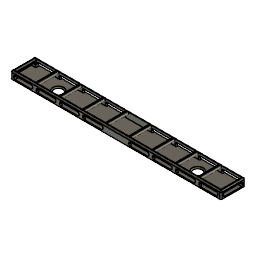
Velcro tie holder (Autodesk Fusion 360 design; units mm, degrees)
part number: 2026-08-08-13-01-59-133
Autodesk Fusion 360 part; units mm, degrees
note: some values were not read from the file. Set by a fixed rule: which face or edge a step refers to.
sketch "Sketch1" plane through (0, 0, 0) normal (0, 0, 1) x (1, 0, 0)
  line L0 (0, 0) -> (20, 0)
  line L1 (20, 0) -> (20, 20)
  line L2 (20, 20) -> (0, 20)
  line L3 (0, 20) -> (0, 0)
  dimension "d1" = 20
  dimension "d2" = 20
  constraint horizontal L0
  constraint vertical L1
  constraint horizontal L2
  constraint vertical L3
  constraint coincident L0.start L3.end
  measures "d1" distance of L0.start L0.end
  measures "d2" distance of L0.start L2.end
extrude "Extrude1" add sketch "Sketch1" along normal blind 1 makes body 1
extrude "Extrude2" add 1 faces at (6.6667, 13.3333, 1) along direction (0, 0, 1) blind 4 thin wall 1 inside on bodies 1 bodies 1
shell "Shell1" thickness 1 removed faces 2 at (6.6667, 0, 1.6667) at (7, 1, 2.3333) on bodies 1
shell "Shell2" thickness 1 removed faces 2 at (20, 6.6667, 1.6667) at (19, 13, 3.3333) on bodies 1
shell "Shell3" thickness 1 removed faces 2 at (0, 13.3333, 1.6667) at (1, 13, 3.3333) on bodies 1
shell "Shell4" thickness 1 removed faces 2 at (13.3333, 20, 1.6667) at (7, 19, 2) on bodies 1
hole "Hole1" at (10, 10, 1) direction (0, 0, -1) diameter 4.5 depth 7 tip angle 180 countersink diameter 8.95 countersink angle 82 bodies 1
copy_body "CopyPasteBodies1" bodies 1 makes body 2
move_body "Move1" bodies 2 to x (1, 0, 0) y (0, 1, 0) z (0, 0, 1) at (19, 0, 0)
delete_face "DeleteFace1" 1 faces at (29.2086, 5.82, 0.6667) on bodies 2
copy_body "CopyPasteBodies2" bodies 2 makes body 3
move_body "Move2" bodies 3 to x (1, 0, 0) y (0, 1, 0) z (0, 0, 1) at (-38, 0, 0)
combine "Combine1" operation add target body 2 tool bodies 3 1
copy_body "CopyPasteBodies3" bodies 2 makes body 4
move_body "Move3" bodies 4 to x (1, 0, 0) y (0, 1, 0) z (0, 0, 1) at (57, 0, 0)
copy_body "CopyPasteBodies4" bodies 2 makes body 5
move_body "Move4" bodies 5 to x (1, 0, 0) y (0, 1, 0) z (0, 0, 1) at (-57, 0, 0)
delete_face "DeleteFace2" 1 faces at (10.2086, 5.82, 0.6667) on bodies 2
combine "Combine2" operation add target body 4 tool bodies 2 5
move_face "OffsetFaces1" offset 1 1 faces at (19.6667, 0.3333, 5) on bodies 4
move_face "OffsetFaces6" offset 1 8 faces at (95, 19.3333, 2) (95.3333, 19, 3) (95.6667, 1, 3) (95, 0.6667, 3) (-75.3333, 1, 3) (-75, 0.3333, 3) (-75.6667, 19, 3) (-75, 19.6667, 2) on bodies 4
move_face "OffsetFaces7" offset 1 1 faces at (-75, 7.3333, 5.3333) on bodies 4
move_face "OffsetFaces8" offset 1 1 faces at (95, 12.6667, 5.3333) on bodies 4
move_face "OffsetFaces9" offset 3 2 faces at (13, 0.3333, 4) (13, 19.3333, 4) on bodies 4
move_face "OffsetFaces10" offset 0.5 3 faces at (-57, 19.3333, 2) (-56.6667, 19, 3) (-56, 19.3333, 2) on bodies 4
move_face "OffsetFaces11" offset 0.5 15 faces at (-38, 19.6667, 2) (-37.6667, 19, 3) (-37, 19.6667, 2) (-18.6667, 19, 3) (-18, 19.6667, 2) (-19, 19.6667, 2) (38, 19.6667, 2) (38.3333, 19, 3) (39, 19.6667, 2) (58, 19.3333, 2) (57.3333, 19, 3) (57, 19.3333, 2) (76, 19.6667, 2) (76.3333, 19, 3) (77, 19.6667, 2) on bodies 4
move_face "OffsetFaces12" offset 0.5 18 faces at (77, 0.3333, 3) (76.6667, 1, 3) (76, 0.3333, 3) (57, 0.6667, 3) (57.6667, 1, 3) (58, 0.3333, 2) (39, 0.3333, 3) (38.6667, 1, 3) (38, 0.3333, 3) (-19, 0.3333, 3) (-18.3333, 1, 3) (-18, 0.3333, 3) (-37, 0.3333, 3) (-37.3333, 1, 3) (-38, 0.3333, 3) (-56, 0.3333, 2) (-56.3333, 1, 3) (-57, 0.6667, 3) on bodies 4
move_face "OffsetFaces13" offset 0.5 18 faces at (-62.8333, 19, 5.3333) (-49.8333, 19, 5.3333) (-30.8333, 19, 5.3333) (-11.8333, 19, 5.3333) (7, 19, 2) (31.8333, 19, 5.3333) (45.1667, 19, 5.3333) (64.1667, 19, 5.3333) (82.8333, 19, 5.3333) (-62.8333, 1, 5.3333) (-44.1667, 1, 5.3333) (-25.1667, 1, 5.3333) (-11.8333, 1, 5.3333) (13, 1, 2) (31.8333, 1, 5.3333) (50.8333, 1, 5.3333) (69.8333, 1, 5.3333) (82.8333, 1, 5.3333) on bodies 4
move_face "OffsetFaces14" offset 0.5 16 faces at (77, 12.8333, 4.6667) (58, 7.1667, 4.6667) (39, 12.8333, 4.6667) (20, 12.8333, 4.6667) (1, 7.1667, 4.6667) (-18, 12.8333, 4.6667) (-37, 12.8333, 4.6667) (-56, 7.1667, 4.6667) (-57, 7.1667, 4.6667) (-38, 12.8333, 4.6667) (-19, 12.8333, 4.6667) (0, 7.1667, 4.6667) (19, 12.8333, 4.6667) (38, 12.8333, 4.6667) (57, 7.1667, 4.6667) (76, 12.8333, 4.6667) on bodies 4
fillet "Fillet1" radius 1 4 edges at (96, 10, 6) (10, 0, 6) (10, 20, 6) (-76, 10, 6) on bodies 4
fillet "Fillet2" radius 1 2 edges at (-76, 20, 2.5) (-75.7071, 19.7071, 5.7071) on bodies 4
fillet "Fillet3" radius 1 2 edges at (-76, 0, 2.5) (-75.7071, 0.2929, 5.7071) on bodies 4
fillet "Fillet4" radius 1 4 edges at (96, 0, 2.5) (95.7071, 0.2929, 5.7071) (96, 20, 2.5) (95.7071, 19.7071, 5.7071) on bodies 4
move_face "OffsetFaces15" offset 0.5 28 faces at (-57.5, 1, 3) (-38.5, 0.5, 3) (-19.5, 1, 2) (0, 1, 3) (37.5, 0.5, 3) (56.5, 0.5, 2) (75.5, 0.5, 3) (75.5, 19.5, 2) (56.5, 19.5, 3) (37.5, 19.5, 2) (0, 19, 2) (-19.5, 19.5, 2) (-38.5, 19.5, 2) (-57.5, 19, 2) (-55.5, 0.5, 2) (-36.5, 1, 2) (-17.5, 0.5, 3) (20, 1, 2) (39.5, 1, 2) (58.5, 0.5, 2) (77.5, 1, 2) (77.5, 19.5, 2) (58.5, 19, 2) (39.5, 19.5, 2) (20, 19.5, 2) (-17.5, 19.5, 2) (-36.5, 19.5, 2) (-55.5, 19.5, 3) on bodies 4
move_face "OffsetFaces16" offset 0.5 16 faces at (-57.5, 7.1667, 4.6667) (-38.5, 12.8333, 4.6667) (-19.5, 12.8333, 4.6667) (-0.5, 7.1667, 4.6667) (18.5, 12.8333, 4.6667) (37.5, 12.8333, 4.6667) (56.5, 7.1667, 4.6667) (75.5, 12.8333, 4.6667) (77.5, 12.8333, 4.6667) (58.5, 7.1667, 4.6667) (39.5, 12.8333, 4.6667) (20.5, 12.8333, 4.6667) (1.5, 7.1667, 4.6667) (-17.5, 12.8333, 4.6667) (-36.5, 12.8333, 4.6667) (-55.5, 7.1667, 4.6667) on bodies 4
move_face "OffsetFaces17" offset 0.5 1 faces at (-74, 12.6667, 5.3333) on bodies 4
move_face "OffsetFaces18" offset 0.5 1 faces at (94, 7.3333, 5.3333) on bodies 4
fillet "Fillet5" radius 1 1 edges at (-17, 0.75, 4) on bodies 4
fillet "Fillet6" radius 1 71 edges at (-0.5, 0.75, 4) (-20, 0.75, 4) (-39, 0.75, 4) (-58, 0.75, 4) (-0.5, 0.75, 1) (-17, 0.75, 1) (-20, 0.75, 1) (-36, 0.75, 1) (-36, 0.75, 4) (-39, 0.75, 1) (-55, 0.75, 1) (-55, 0.75, 4) (-73.5, 0.75, 4) (-73.5, 1, 1) (-58, 0.75, 1) (-58, 19.25, 1) (-73.5, 19.25, 4) (-74.75, 2, 1) (-74.75, 2, 4) (-74.75, 18, 4) (-74.75, 18, 1) (-73.5, 19, 1) (-58, 19.25, 4) (-39, 19.25, 4) (-39, 19.25, 1) (-55, 19.25, 1) (-55, 19.25, 4) (-20, 19.25, 1) (-20, 19.25, 4) (-36, 19.25, 1) (-36, 19.25, 4) (-17, 19.25, 4) (-17, 19.25, 1) (-0.5, 19.25, 1) (-0.5, 19.25, 4) (37, 19.25, 1) (56, 19.25, 1) (37, 19.25, 4) (20.5, 19.25, 1) (20.5, 19.25, 4) (40, 19.25, 4) (40, 19.25, 1) (56, 19.25, 4) (75, 19.25, 4) (75, 19.25, 1) (59, 19.25, 1) (59, 19.25, 4) (78, 19.25, 4) (78, 19.25, 1) (93.5, 19, 1) (93.5, 19.25, 4) (94.75, 2, 4) (94.75, 2, 1) (94.75, 18, 1) (94.75, 18, 4) (78, 0.75, 1) (78, 0.75, 4) (93.5, 0.75, 4) (93.5, 1, 1) (75, 0.75, 1) (75, 0.75, 4) (59, 0.75, 1) (59, 0.75, 4) (40, 0.75, 4) (40, 0.75, 1) (56, 0.75, 1) (56, 0.75, 4) (37, 0.75, 1) (37, 0.75, 4) (20.5, 0.75, 1) (20.5, 0.75, 4) on bodies 4
fillet "Fillet7" radius 1 4 edges at (-58, 10, 6) (-58, 10, 4) (-55, 10, 4) (-55, 10, 6) on bodies 4
fillet "Fillet8" radius 1 1 edges at (-73.5, 10, 6) on bodies 4
fillet "Fillet9" radius 1 29 edges at (-39, 10, 6) (-36, 10, 6) (-20, 10, 6) (-17, 10, 6) (-1, 10, 6) (2, 10, 6) (18, 10, 6) (21, 10, 6) (37, 10, 6) (40, 10, 6) (56, 10, 6) (59, 10, 6) (75, 10, 6) (78, 10, 6) (93.5, 10, 6) (78, 10, 4) (59, 10, 4) (40, 10, 4) (21, 10, 4) (-1, 10, 4) (2, 10, 4) (-17, 10, 4) (-36, 10, 4) (-39, 10, 4) (-20, 10, 4) (18, 10, 4) (37, 10, 4) (56, 10, 4) (75, 10, 4) on bodies 4
delete_face "DeleteFace3" [suppressed]
move_face "OffsetFaces2" [suppressed]
move_face "OffsetFaces3" [suppressed]
move_face "OffsetFaces4" [suppressed]
move_face "OffsetFaces5" [suppressed]
